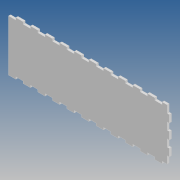
# Autodesk Inventor part: 000.102 - Left wall
Saved by Autodesk Inventor 2020 (Build 240168000, 168)
## iProperties
Created: 2021-06-28
Part Number: 000.102 - Left wall
Material: Типовые
Document SubType Name: Modeling
Designer: Петров Иван
Mass: 45.84 g
Surface Area: 327.14 cm^2
Volume: 45.84 cm^3
Density: 1 g/cm^3
Appearance: По умолчанию
Author: Петров Иван
Autodesk Inventor part; units mm, degrees
ref_plane "YZ Plane" through (0, 0, 0) normal (1, 0, 0) x (0, 1, 0)
ref_plane "XZ Plane" through (0, 0, 0) normal (0, 1, 0) x (-1, 0, 0)
ref_plane "XY Plane" through (0, 0, 0) normal (0, 0, 1) x (1, 0, 0)
sketch "Эскиз1" plane through (0, 0, 0) normal (0, 0, 1) x (1, 0, 0)
  line L0 (0, 0) -> (10, 0)
  line L1 (10, 0) -> (10, 3)
  line L2 (10, 3) -> (0, 3)
  line L3 (0, 3) -> (0, 0)
  dimension "d0" = 10
  dimension "d1" = 3
  constraints: 8 end point, 2 parallel, 1 horizontal, 1 perpendicular
  measures "d0" distance of L2.end L1.end
  measures "d1" distance of L1.end L0.end
extrude "Выдавливание1" add sketch "Эскиз1" along normal blind 3
pattern_linear "Прямоуг.массив1" count 11 spacing 20 along (1, 0, 0) of "Выдавливание1"
sketch "Эскиз2" plane through (0, 0, 3) normal (0, 0, 1) x (1, 0, 0)
  line L0 (0, 3) -> (0, 0) projected
  line L1 (0, 3) -> (220, 3)
  line L2 (220, 3) -> (220, 73)
  line L3 (220, 73) -> (0, 73)
  line L4 (0, 73) -> (0, 3)
  line L5 (210, 0) -> (210, 3) projected
  dimension "d8" = 70
  dimension "d11" = 10
  constraints: 8 end point, 2 parallel, 1 horizontal, 1 perpendicular
  measures "d8" distance of L1.end L2.end
  measures "d11" distance between parallel lines of L2 L5
extrude "Выдавливание2" add sketch "Эскиз2" against normal blind 3
sketch "Эскиз3" plane through (0, 0, 3) normal (0, 0, 1) x (1, 0, 0)
  line L0 (0, 73) -> (220, 73) projected
  line L1 (220, 73) -> (217, 73)
  line L2 (217, 73) -> (217, 63)
  line L3 (217, 63) -> (220, 63)
  line L4 (220, 63) -> (220, 73)
  point P0 (0, 0)
  dimension "d12" = 3
  dimension "d13" = 10
  constraints: 8 end point, 2 parallel, 1 horizontal, 1 perpendicular
  measures "d12" distance of L3.end L2.end
  measures "d13" distance of L2.end L1.end
extrude "Выдавливание3" cut sketch "Эскиз3" against normal blind 10
pattern_linear "Прямоуг.массив2" count 4 spacing 20 along (0, -1, 0) of "Выдавливание3"
sketch "Эскиз4" plane through (0, 0, 3) normal (0, 0, 1) x (1, 0, 0)
  line L0 (0, 73) -> (217, 73) projected
  line L1 (0, 73) -> (10, 73)
  line L2 (10, 73) -> (10, 70)
  line L3 (10, 70) -> (0, 70)
  line L4 (0, 70) -> (0, 73)
  point P0 (0, 0)
  dimension "d19" = 10
  dimension "d20" = 3
  constraints: 8 end point, 2 parallel, 1 horizontal, 1 perpendicular
  measures "d19" distance of L2.end L3.end
  measures "d20" distance of L1.end L2.end
extrude "Выдавливание4" cut sketch "Эскиз4" against normal blind 10
pattern_linear "Прямоуг.массив3" count 11 spacing 20 along (1, 0, 0) of "Выдавливание4"
